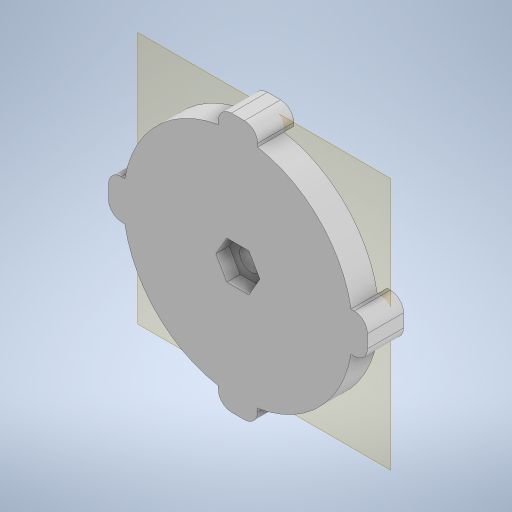
# Autodesk Inventor part: dol
Saved by Autodesk Inventor 2023 (Build 270158000, 158)
## iProperties
Created: 2023-08-20
Part Number: dol
Material: Ogólny
Document SubType Name: Modeling
Designer: Kamil
Density: 1 g/cm^3
Appearance: Domyślna
Author: Kamil
Autodesk Inventor part; units mm, degrees
ref_plane "YZ Plane" through (0, 0, 0) normal (1, 0, 0) x (0, 1, 0)
ref_plane "XZ Plane" through (0, 0, 0) normal (0, 1, 0) x (-1, 0, 0)
ref_plane "XY Plane" through (0, 0, 0) normal (0, 0, 1) x (1, 0, 0)
ref_plane "Płaszczyzna konstrukcyjna1" through (0, 0, 0) normal (0, 0, 1) x (1, 0, 0)
sketch "Szkic1" plane through (0, 0, 0) normal (0, 0, 1) x (1, 0, 0)
  circle A0 centre (0, 0) radius 17.5 projected
  line L0 (17.7409, 3) -> (17.4439, 3) projected
  arc A1 (17.4439, -3) -> (17.4439, 3) centre (0, 0) ccw projected
  line L1 (17.4439, -3) -> (17.7409, -3) projected
  line L2 (19.7409, -1) -> (19.7409, 1) projected
  line L3 (3, -17.7409) -> (3, -17.4439) projected
  arc A2 (-3, -17.4439) -> (3, -17.4439) centre (0, 0) ccw projected
  line L4 (-3, -17.4439) -> (-3, -17.7409) projected
  line L5 (-1, -19.7409) -> (1, -19.7409) projected
  circle A3 centre (0, 0) radius 1.75 projected
  line L6 (17.7409, -3) -> (5, -3) projected
  line L7 (3, -5) -> (3, -17.7409) projected
  line L8 (1, -19.7409) -> (-1, -19.7409) projected
  line L9 (-3, -17.7409) -> (-3, -5) projected
  line L10 (-5, -3) -> (-17.7409, -3) projected
  line L11 (-19.7409, -1) -> (-19.7409, 1) projected
  line L12 (-17.7409, 3) -> (-5, 3) projected
  line L13 (-3, 5) -> (-3, 17.7409) projected
  line L14 (-1, 19.7409) -> (1, 19.7409) projected
  line L15 (3, 17.7409) -> (3, 3) projected
  line L16 (3, 3) -> (17.7409, 3) projected
  line L17 (19.7409, 1) -> (19.7409, -1) projected
  arc A4 (-3, -17.7409) -> (-1, -19.7409) centre (-1, -17.7409) ccw projected
  arc A5 (1, -19.7409) -> (3, -17.7409) centre (1, -17.7409) ccw projected
  arc A6 (19.7409, 1) -> (17.7409, 3) centre (17.7409, 1) ccw projected
  arc A7 (17.7409, -3) -> (19.7409, -1) centre (17.7409, -1) ccw projected
  arc A8 (5, -3) -> (3, -5) centre (5, -5) ccw projected
  arc A9 (1, -19.7409) -> (3, -17.7409) centre (1, -17.7409) ccw projected
  arc A10 (-3, -17.7409) -> (-1, -19.7409) centre (-1, -17.7409) ccw projected
  arc A11 (-3, -5) -> (-5, -3) centre (-5, -5) ccw projected
  arc A12 (-19.7409, -1) -> (-17.7409, -3) centre (-17.7409, -1) ccw projected
  arc A13 (-17.7409, 3) -> (-19.7409, 1) centre (-17.7409, 1) ccw projected
  arc A14 (-5, 3) -> (-3, 5) centre (-5, 5) ccw projected
  arc A15 (-1, 19.7409) -> (-3, 17.7409) centre (-1, 17.7409) ccw projected
  arc A16 (3, 17.7409) -> (1, 19.7409) centre (1, 17.7409) ccw projected
  arc A17 (19.7409, 1) -> (17.7409, 3) centre (17.7409, 1) ccw projected
  arc A18 (17.7409, -3) -> (19.7409, -1) centre (17.7409, -1) ccw projected
  point P0 (3, -19.7409)
  point P1 (-3, -19.7409)
  point P2 (17.2409, 3)
  point P3 (3, 17.2409)
  point P4 (-3, 17.2409)
  point P5 (-17.2409, 3)
  point P6 (-17.2409, -3)
  point P7 (-3, -17.2409)
  point P8 (3, -17.2409)
  point P9 (17.2409, -3)
extrude "Wyciągnięcie proste1" add sketch "Szkic1" along normal blind 4 contours A0 L6 A8 L7 L9 A11 L10 L12 A14 L13 L15 L16 | A0 L16 A1 L6 | L16 L15 A0 | A0 L7 A8 L6 | A0 L13 A15 L14 A16 L15 | L0 A6 L2 A7 L1 A1 | L7 A2 L9 A0 | L13 A14 L12 A0 | A0 L10 A11 L9 | A0 L10 A12 L11 A13 L12 | A3
sketch "Szkic2" plane through (0, 0, 0) normal (0, 0, -1) x (-1, 0, 0)
  circle A0 centre (0, 0) radius 17.5 projected
  circle A1 centre (0, 0) radius 1.75 projected
  line L0 (-17.7409, -3) -> (-5, -3) projected
  line L1 (-3, -5) -> (-3, -17.7409) projected
  line L2 (-1, -19.7409) -> (1, -19.7409) projected
  line L3 (3, -17.7409) -> (3, -5) projected
  line L4 (5, -3) -> (17.7409, -3) projected
  line L5 (19.7409, -1) -> (19.7409, 1) projected
  line L6 (17.7409, 3) -> (5, 3) projected
  line L7 (3, 5) -> (3, 17.7409) projected
  line L8 (1, 19.7409) -> (-1, 19.7409) projected
  line L9 (-3, 17.7409) -> (-3, 3) projected
  line L10 (-3, 3) -> (-17.7409, 3) projected
  line L11 (-19.7409, 1) -> (-19.7409, -1) projected
  circle A2 centre (0, 0) radius 17.7
  arc A3 (-17.7409, 3) -> (-19.7409, 1) centre (-17.7409, 1) ccw projected
  arc A4 (-19.7409, -1) -> (-17.7409, -3) centre (-17.7409, -1) ccw projected
  arc A5 (-3, -5) -> (-5, -3) centre (-5, -5) ccw projected
  arc A6 (-3, -17.7409) -> (-1, -19.7409) centre (-1, -17.7409) ccw projected
  arc A7 (1, -19.7409) -> (3, -17.7409) centre (1, -17.7409) ccw projected
  arc A8 (5, -3) -> (3, -5) centre (5, -5) ccw projected
  arc A9 (17.7409, -3) -> (19.7409, -1) centre (17.7409, -1) ccw projected
  arc A10 (19.7409, 1) -> (17.7409, 3) centre (17.7409, 1) ccw projected
  arc A11 (3, 5) -> (5, 3) centre (5, 5) ccw projected
  arc A12 (3, 17.7409) -> (1, 19.7409) centre (1, 17.7409) ccw projected
  arc A13 (-1, 19.7409) -> (-3, 17.7409) centre (-1, 17.7409) ccw projected
  point P0 (17.4439, 3)
  point P1 (17.4439, -3)
  point P2 (3, -17.4439)
  point P3 (-3, -17.4439)
  point P4 (-17.4439, -3)
  point P5 (-17.4439, 3)
  point P6 (-3, 17.4439)
  point P7 (3, 17.4439)
  dimension "d2" = 0.2
  constraints: 1 centre point
  measures "d2" radial gap between concentric circles of A0 A2
extrude "Wyciągnięcie proste2" add sketch "Szkic2" along normal blind 1.5 contours L6 A11 L7 A0 | A0 L7 A2 L6 | L4 A2 L3 A0 | A0 L3 A8 L4 | L6 A10 L5 A9 L4 A2 | L9 L10 A0 | A0 L10 A2 L9 | A2 L9 A13 L8 A12 L7 | L1 A2 L0 A0 | A0 L0 A5 L1 | L3 A7 L2 A6 L1 A2 | A2 L0 A4 L11 A3 L10
sketch "Szkic3" plane through (0, 0, 4) normal (0, 0, 1) x (1, 0, 0)
  arc A0 (17.2409, 3) -> (3, 17.2409) centre (0, 0) ccw projected
  line L0 (17.4439, 3) -> (17.2409, 3) projected
  arc A1 (17.4439, 3) -> (3, 17.4439) centre (0, 0) ccw projected
  line L1 (3, 17.2409) -> (3, 17.4439) projected
  arc A2 (3, -17.2409) -> (17.2409, -3) centre (0, 0) ccw projected
  line L2 (3, -17.4439) -> (3, -17.2409) projected
  arc A3 (3, -17.4439) -> (17.4439, -3) centre (0, 0) ccw projected
  line L3 (17.2409, -3) -> (17.4439, -3) projected
  arc A4 (-17.2409, -3) -> (-3, -17.2409) centre (0, 0) ccw projected
  line L4 (-17.4439, -3) -> (-17.2409, -3) projected
  arc A5 (-17.4439, -3) -> (-3, -17.4439) centre (0, 0) ccw projected
  line L5 (-3, -17.2409) -> (-3, -17.4439) projected
  arc A6 (-3, 17.2409) -> (-17.2409, 3) centre (0, 0) ccw projected
  line L6 (-3, 17.4439) -> (-3, 17.2409) projected
  arc A7 (-3, 17.4439) -> (-17.4439, 3) centre (0, 0) ccw projected
  line L7 (-17.2409, 3) -> (-17.4439, 3) projected
extrude "Wyciągnięcie proste3" cut sketch "Szkic3" against normal through all
sketch "Szkic4" plane through (0, 0, -1.5) normal (0, 0, -1) x (-1, 0, 0)
  arc A0 (17.2409, 3) -> (3, 17.2409) centre (0, 0) ccw projected
  line L0 (3, 17.2409) -> (3, 5) projected
  arc A1 (3, 5) -> (5, 3) centre (5, 5) ccw projected
  line L1 (5, 3) -> (17.2409, 3) projected
  arc A2 (-3, 17.2409) -> (-17.2409, 3) centre (0, 0) ccw projected
  line L2 (-17.2409, 3) -> (-3, 3) projected
  line L3 (-3, 3) -> (-3, 17.2409) projected
  arc A3 (-17.2409, -3) -> (-3, -17.2409) centre (0, 0) ccw projected
  line L4 (-3, -17.2409) -> (-3, -5) projected
  arc A4 (-3, -5) -> (-5, -3) centre (-5, -5) ccw projected
  line L5 (-5, -3) -> (-17.2409, -3) projected
  arc A5 (3, -17.2409) -> (17.2409, -3) centre (0, 0) ccw projected
  line L6 (17.2409, -3) -> (5, -3) projected
  arc A6 (5, -3) -> (3, -5) centre (5, -5) ccw projected
  line L7 (3, -5) -> (3, -17.2409) projected
extrude "Wyciągnięcie proste4" cut sketch "Szkic4" against normal up to surface (1.5 mm away)
sketch "Szkic5" plane through (0, 0, 0) normal (0, 0, 1) x (1, 0, 0)
  line L0 (-3, -17.7409) -> (-3, -17.4439) projected
  arc A0 (-3, -17.7409) -> (-1, -19.7409) centre (-1, -17.7409) ccw projected
  line L1 (1, -19.7409) -> (-1, -19.7409) projected
  arc A1 (1, -19.7409) -> (3, -17.7409) centre (1, -17.7409) ccw projected
  line L2 (3, -17.4439) -> (3, -17.7409) projected
  arc A2 (-3, -17.4439) -> (3, -17.4439) centre (0, 0) ccw projected
extrude "Wyciągnięcie proste5" add sketch "Szkic5" along normal up to surface (4 mm away)
sketch "Szkic6" plane through (0, 0, 4) normal (0, 0, 1) x (1, 0, 0)
  circle A0 centre (0, 0) radius 2.9
  line L0 (-1.6743, -2.9) -> (-3.3486, 0)
  line L1 (-3.3486, 0) -> (-1.6743, 2.9)
  line L2 (-1.6743, 2.9) -> (1.6743, 2.9)
  line L3 (1.6743, 2.9) -> (3.3486, 0)
  line L4 (3.3486, 0) -> (1.6743, -2.9)
  line L5 (1.6743, -2.9) -> (-1.6743, -2.9)
  point P0 (0, -2.9)
  dimension "d11" = 5.8
  constraints: 12 end point, 2 coincident, 1 midpoint, 1 vertical alignment, 15 other
extrude "Wyciągnięcie proste6" cut sketch "Szkic6" against normal blind 2
sketch "Szkic7" plane through (0, 0, 2) normal (0, 0, 1) x (1, 0, 0)
  line L0 (1.6743, 2.9) -> (3.3486, 0) projected
  line L1 (3.3486, 0) -> (1.6743, -2.9) projected
  line L2 (1.6743, -2.9) -> (-1.6743, -2.9) projected
  line L3 (-1.6743, -2.9) -> (-3.3486, 0) projected
  line L4 (-3.3486, 0) -> (-1.6743, 2.9) projected
  line L5 (-1.6743, 2.9) -> (1.6743, 2.9) projected
  line L6 (-3, -17.2409) -> (-3, -17.7409) projected
  arc A0 (-3, -17.7409) -> (-1, -19.7409) centre (-1, -17.7409) ccw projected
  line L7 (1, -19.7409) -> (-1, -19.7409) projected
  arc A1 (1, -19.7409) -> (3, -17.7409) centre (1, -17.7409) ccw projected
  line L8 (3, -17.2409) -> (3, -17.7409) projected
  arc A2 (3, -17.2409) -> (17.2409, -3) centre (0, 0) ccw projected
  line L9 (17.2409, -3) -> (17.7409, -3) projected
  arc A3 (17.7409, -3) -> (19.7409, -1) centre (17.7409, -1) ccw projected
  line L10 (19.7409, -1) -> (19.7409, 1) projected
  arc A4 (19.7409, 1) -> (17.7409, 3) centre (17.7409, 1) ccw projected
  line L11 (17.7409, 3) -> (17.2409, 3) projected
  arc A5 (17.2409, 3) -> (3, 17.2409) centre (0, 0) ccw projected
  line L12 (3, 17.2409) -> (3, 17.7409) projected
  arc A6 (3, 17.7409) -> (1, 19.7409) centre (1, 17.7409) ccw projected
  line L13 (1, 19.7409) -> (-1, 19.7409) projected
  arc A7 (-1, 19.7409) -> (-3, 17.7409) centre (-1, 17.7409) ccw projected
  line L14 (-3, 17.7409) -> (-3, 17.2409) projected
  arc A8 (-3, 17.2409) -> (-17.2409, 3) centre (0, 0) ccw projected
  line L15 (-17.2409, 3) -> (-17.7409, 3) projected
  arc A9 (-17.7409, 3) -> (-19.7409, 1) centre (-17.7409, 1) ccw projected
  line L16 (-19.7409, 1) -> (-19.7409, -1) projected
  arc A10 (-19.7409, -1) -> (-17.7409, -3) centre (-17.7409, -1) ccw projected
  line L17 (-17.7409, -3) -> (-17.2409, -3) projected
  arc A11 (-17.2409, -3) -> (-3, -17.2409) centre (0, 0) ccw projected
  circle A12 centre (0, 0) radius 1.75
  dimension "d14" = 3.5
  constraints: 1 centre point, 1 coincident
  measures "d14" diameter of A12
extrude "Wyciągnięcie proste7" cut sketch "Szkic7" against normal through all contours A12
sketch "Szkic8" plane through (0, 0, 0) normal (0, 0, -1) x (-1, 0, 0)
  circle A0 centre (0, 0) radius 1.75 projected
  arc A1 (-17.2409, -3) -> (-3, -17.2409) centre (0, 0) ccw projected
  line L0 (-3, -17.4439) -> (-3, -17.2409) projected
  arc A2 (-3, -17.4439) -> (3, -17.4439) centre (0, 0) ccw projected
  line L1 (3, -17.2409) -> (3, -17.4439) projected
  arc A3 (3, -17.2409) -> (17.2409, -3) centre (0, 0) ccw projected
  line L2 (17.4439, -3) -> (17.2409, -3) projected
  arc A4 (17.4439, -3) -> (17.4439, 3) centre (0, 0) ccw projected
  line L3 (17.2409, 3) -> (17.4439, 3) projected
  arc A5 (17.2409, 3) -> (3, 17.2409) centre (0, 0) ccw projected
  line L4 (3, 17.4439) -> (3, 17.2409) projected
  arc A6 (3, 17.4439) -> (-3, 17.4439) centre (0, 0) ccw projected
  line L5 (-3, 17.2409) -> (-3, 17.4439) projected
  arc A7 (-3, 17.2409) -> (-17.2409, 3) centre (0, 0) ccw projected
  line L6 (-17.4439, 3) -> (-17.2409, 3) projected
  arc A8 (-17.4439, 3) -> (-17.4439, -3) centre (0, 0) ccw projected
  line L7 (-17.2409, -3) -> (-17.4439, -3) projected
  circle A9 centre (0, 0) radius 17.5
  point P0 (-3, -17.2409)
  point P1 (-17.2409, 3)
  point P2 (3, 17.2409)
  point P3 (17.2409, -3)
  dimension "d17" = 35
  constraints: 1 centre point, 1 coincident
  measures "d17" diameter of A9
extrude "Wyciągnięcie proste8" add sketch "Szkic8" along normal up to surface (1.5 mm away) contours L7 A8 L6 A9 | A9 L1 A2 L0 | L5 A6 L4 A9 | A9 L3 A4 L2
